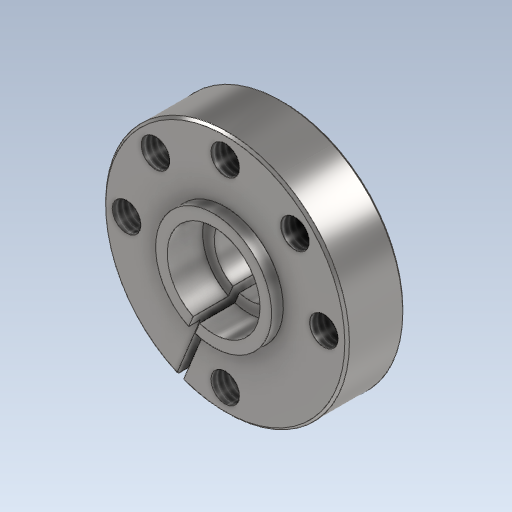
# Autodesk Inventor part: ClampHorn
Saved by Autodesk Inventor 2020.4 (Build 244396000, 396)
## iProperties
Part Number: ClampHorn
Material: ステンレス鋼 AISI 304
Document SubType Name: Modeling
Designer: Masato Kubotera
Density: 8 g/cm^3
Appearance: 半つや出し
Catalog Web Link: https://kondo-robot.com/product/02031
Description: ReaedyMade
Author: Masato Kubotera
Autodesk Inventor part; units mm, degrees
ref_plane "YZ Plane" through (0, 0, 0) normal (1, 0, 0) x (0, 1, 0)
ref_plane "XZ Plane" through (0, 0, 0) normal (0, 1, 0) x (-1, 0, 0)
ref_plane "XY Plane" through (0, 0, 0) normal (0, 0, 1) x (1, 0, 0)
sketch "スケッチ1" plane through (0, 0, 0) normal (0, 1, 0) x (-1, 0, 0)
  line L0 (-3, 0) -> (-3, 4.25)
  line L1 (-3, 4.25) -> (-4, 4.25)
  line L2 (-4, 4.25) -> (-4, 7.3)
  line L3 (-4, 7.3) -> (-5, 7.3)
  line L4 (-5, 7.3) -> (-5, 6.3)
  line L5 (-5, 6.3) -> (-10.5, 6.3)
  line L6 (-10.5, 6.3) -> (-10.5, 1.3)
  line L7 (-10.5, 1.3) -> (-4, 1.3)
  line L8 (-4, 1.3) -> (-4, 0)
  line L9 (-4, 0) -> (-3, 0)
  line L10 (0, -1.46) -> (0, 8.76) projected
  line L11 (-8.5, 6.3) -> (-8.5, 1.3) construction
  point P0 (0, 0)
  dimension "d0" = 6
  dimension "d1" = 8
  dimension "d2" = 8
  dimension "d3" = 10
  dimension "d4" = 5
  dimension "d5" = 1
  dimension "d6" = 1.3
  dimension "d7" = 3.05
  dimension "d8" = 21
  dimension "d9" = 17
  constraints: 22 end point, 9 perpendicular, 3 point on line, 2 vertical
  measures "d0" diameter of L0.start L10
  measures "d1" diameter of L8.end L10
  measures "d2" diameter of L2.end L10
  measures "d3" diameter of L3.end L10
  measures "d4" distance of L5.end L6.end
  measures "d5" distance of L3.end L4.end
  measures "d6" distance of L7.end L8.end
  measures "d7" distance of L1.end L2.end
  measures "d8" diameter of L6.end L10
  measures "d9" diameter of L11.start L10
revolve "回転1" add sketch "スケッチ1" angle 360 about axis through (0, 0, -10) along (0, 0, 1)
sketch "スケッチ2" plane through (0, 0, 6.3) normal (0, 0, 1) x (1, 0, 0)
  line L0 (-0.2782, 0.1124) -> (0.2782, -0.1124)
  line L1 (0.2782, -0.1124) -> (-3.6552, -9.8478)
  line L2 (-3.6552, -9.8478) -> (-4.2115, -9.623)
  line L3 (-4.2115, -9.623) -> (-0.2782, 0.1124)
  circle A0 centre (0, 0) radius 10.5 projected
  line L4 (0, -14.7) -> (0, 14.7) projected
  point P0 (8.5, 0)
  point P1 (8.5, 0)
  point P2 (8.5, 0)
  point P3 (8.5, 0)
  point P4 (0, -0.8008)
  point P5 (-4.2099, -9.6191)
  point P6 (-3.6536, -9.8438)
  dimension "d21" = 0.6
  dimension "d22" = 22
  constraints: 8 end point, 2 coincident, 2 perpendicular, 1 midpoint, 1 parallel, 1 tangent
  measures "d21" distance of L1.end L2.end
  measures "d22" angle of L1 L4
hole "穴1" at (8.5, 0, 6.3) direction (0, 0, -1) diameter 2.459 end through all thread size "M3x0.5" class "6H" standard "ISO Metric profile"
pattern_circular "円形状パターン1" count 8 over 360 about axis through (0, 0, -10) along (0, 0, 1) of "穴1" skipped copies 6 8
extrude "押し出し1" cut sketch "スケッチ2" along normal through all both and the other way through all contours L0 L4 L1 A0 L3
chamfer "面取り1" distance 0.2 angle 45 4 edges at (-5.7466, 8.7879, 6.3) (5.9953, -8.6201, 6.3) (5.9953, -8.6201, 1.3) (-5.7466, 8.7879, 1.3)
